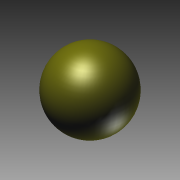
# Autodesk Inventor part: 6005_PART3
Saved by Autodesk Inventor 2011 SP1 (Build 150282100, 282)
## iProperties
Created: 2017-09-09
Part Number: 6005_PART3
Catalog Web Link: www.cadenas.de
Description: -Deep groove ball bearings, single row
Vendor: SKF
Document SubType Name: Modeling
Designer: psAdmin
Manufacturer: SKF
Mass: 0.160817 g
Surface Area: 1.43012 cm^2
Volume: 0.160817 cm^3
Density: 1 g/cm^3
Category: PARTsolutions
Company: SKF
Title: 6005_PART3
Author: Cadenas PARTsolutions
Comments: Deep groove ball bearings, single row
PSOL_IDENT_0: {$CADENAS_DATA\23d-libs\skf\bearings_units_and_housings\ball_bearings\deep_groove_ball_bearings\deep
PSOL_IDENT_1: _groove_ball_bearings_single_row\bb1_001_101.prj},190 {VTYP=3D},{NB=6005_PART3},{LINA=6005_PART3},{N
PSOL_IDENT_2: N=BB1_001_101_PART3},{NOPRJ=TRUE},{DATE=14.07.2017 09:01:20},{GEOMDATE=14.07.2017 08:21:21},{VERSION=
PSOL_IDENT_3: },{LINEID=214610},{LINESUBID=-1},{WBVAR=}  {NB=6005_PART3},{LINA=6005_PART3},{KT=DUMMY},{PRODUCTID=1
PSOL_IDENT_4: 050010005},{DESIGNATION=6005},{DD=25.000},{D=47.000},{B=12.000},{HH=-1000000015047466219876688855040
PSOL_IDENT_5: .000},{DD1=32.000},{DD2=-1000000015047466219876688855040.000},{DD22=-1000000015047466219876688855040
PSOL_IDENT_6: .000},{D1=40.000},{D2=42.200},{BB=-1000000015047466219876688855040.000},{R12=0.6},{R121=0.600},{R122=
PSOL_IDENT_7: 0.600},{LOAD1=11.900},{LOAD2=6.550},{LOAD3=0.275},{SPEED1=32000},{SPEED2=20000},{MASS=0.078},{PITCH=
PSOL_IDENT_8: 36.000},{DW=6.747},{Z=10.000},{II=1.000},{TYPEID=105001},{HELP=3.5},{HELP2=2.4},{DD1ALG=16},{TAXONOM
PSOL_IDENT_9: Y=1},{DESIGN=dgbb1},{MAPPING=BCZ50,DESIGNATION|IRD01,DD|ORD10,D|BCW30,B|ORL64,HH|IRD30,DD1|IRD46,DD2
PSOL_IDENT_10: |IRD43,DD22|ORD30,D1|ORD43,D2|ORL60,BB|ORL03,R121|BCE41,R122|BCC02,LOAD1|BCC16,LOAD2|BCC12,LOAD3|BCC
PSOL_IDENT_11: 43,SPEED1|BCC45,SPEED2|BCM01,MASS|BCD50,PITCH|RBD10,DW|BCN81,Z|BCN80,II},{DESIGNLIST=dgbbrs,dgbb1,dg
PSOL_IDENT_12: bb2rs,dgbb2z,dgbbn1,dgbbz},{YALG=16.00000},{HALG=3.50000},{YALG1=20.00000},{HALG1=3.50000},{PITCH1=3
PSOL_IDENT_13: 6.00000},{DW1=6.74700},{SH=16},{CU=1.0506},{SORT=DD},{PIM=6005}
NT: Deep groove ball bearings, single row
NB: 6005_PART3
NBSYN: $DESIGNATION._PART3
LINA: 6005_PART3
DESIGNATION: 6005
DD: 25.000
D: 47.000
B: 12.000
LOAD1: 11.900
LOAD2: 6.550
LOAD3: 0.275
SPEED1: 32000
SPEED2: 20000
SUPPLIER: SKF
ARTICLENO: 6005_PART3
BOMINFO: 6005_PART3
CREATOR: CADENAS GmbH
Autodesk Inventor part; units mm, degrees
ref_plane "YZ Plane" through (0, 0, 0) normal (1, 0, 0) x (0, 1, 0)
ref_plane "XZ Plane" through (0, 0, 0) normal (0, 1, 0) x (-1, 0, 0)
ref_plane "XY Plane" through (0, 0, 0) normal (0, 0, 1) x (1, 0, 0)
sketch "Sketch_1" plane through (0, 0, 0) normal (0, 0, 1) x (1, 0, 0)
  line L0 (9.3735, 18) -> (2.6265, 18)
  arc A0 (9.3735, 18) -> (2.6265, 18) centre (6, 18) ccw
  line L1 (9.3735, 18) -> (2.6265, 18)
  dimension "d0" = 360
  constraints: 4 end point, 2 point on circle, 1 centre point
revolve "Revolution1" add sketch "Sketch_1" angle 360 about axis through (9.3735, 18, 0) along (1, 0, 0)
body "Solid1"
